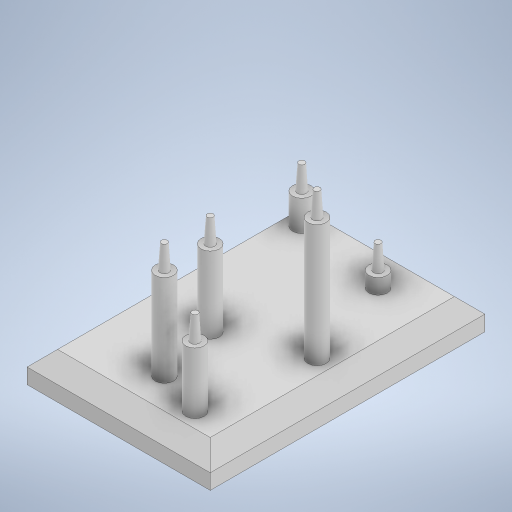
# Autodesk Inventor part: HeadTrackerProMax
Saved by Autodesk Inventor 2024 (Build 280153000, 153)
## iProperties
Created: 2024-11-04
Part Number: HeadTrackerProMax
Material: 一般
Document SubType Name: Modeling
Designer: jerry
Density: 1 g/cm^3
Appearance: 預設
Author: jerry
Autodesk Inventor part; units mm, degrees
ref_plane "YZ Plane" through (0, 0, 0) normal (1, 0, 0) x (0, 1, 0)
ref_plane "XZ Plane" through (0, 0, 0) normal (0, 1, 0) x (-1, 0, 0)
ref_plane "XY Plane" through (0, 0, 0) normal (0, 0, 1) x (1, 0, 0)
sketch "草圖1" plane through (0, 0, 0) normal (0, 1, 0) x (-1, 0, 0)
  line L0 (0, 0) -> (60, 0)
  line L1 (60, 0) -> (60, -90)
  line L2 (60, -90) -> (0, -90)
  line L3 (0, -90) -> (0, 0)
  dimension "d0" = 60
  dimension "d1" = 90
  constraints: 8 end point, 2 parallel, 1 horizontal, 1 perpendicular
  measures "d0" distance of L1.end L2.end
  measures "d1" distance of L0.end L1.end
extrude "擠出1" add sketch "草圖1" along normal blind 10
chamfer "倒角1" distance 5 angle 45 4 edges at (-60, 10, -45) (-30, 10, 0) (0, 10, -45) (-30, 10, -90)
sketch "草圖2" plane through (0, 10, 0) normal (0, 1, 0) x (1, 0, 0)
  line L0 (-60, 0) -> (0, 0) projected
  line L1 (0, 0) -> (-15, 0)
  line L2 (-15, 0) -> (-15, 10)
  line L3 (-15, 10) -> (0, 10)
  line L4 (0, 10) -> (0, 0)
  line L5 (-15, 10) -> (-30, 10)
  line L6 (-30, 10) -> (-30, 15)
  line L7 (-30, 15) -> (-15, 15)
  line L8 (-15, 15) -> (-15, 10)
  line L9 (-30, 15) -> (-35, 15)
  line L10 (-35, 15) -> (-35, 35)
  line L11 (-35, 35) -> (-30, 35)
  line L12 (-30, 35) -> (-30, 15)
  line L13 (-35, 35) -> (-50, 35)
  line L14 (-50, 35) -> (-50, 80)
  line L15 (-50, 80) -> (-35, 80)
  line L16 (-35, 80) -> (-35, 35)
  line L17 (-35, 80) -> (-20, 80)
  line L18 (-20, 80) -> (-20, 75)
  line L19 (-20, 75) -> (-35, 75)
  line L20 (-35, 75) -> (-35, 80)
  line L21 (-20, 75) -> (-10, 75)
  line L22 (-10, 75) -> (-10, 45)
  line L23 (-10, 45) -> (-20, 45)
  line L24 (-20, 45) -> (-20, 75)
  circle A0 centre (-15, 10) radius 3
  circle A1 centre (-30, 15) radius 3
  circle A2 centre (-35, 35) radius 3
  circle A3 centre (-50, 80) radius 3
  circle A4 centre (-20, 75) radius 3
  circle A5 centre (-10, 45) radius 3
  dimension "d7" = 15
  dimension "d8" = 10
  dimension "d9" = 15
  dimension "d10" = 5
  dimension "d11" = 5
  dimension "d12" = 20
  dimension "d13" = 15
  dimension "d14" = 45
  dimension "d15" = 15
  dimension "d16" = 5
  dimension "d17" = 10
  dimension "d18" = 30
  dimension "d19" = 6
  dimension "d20" = 6
  dimension "d21" = 6
  dimension "d22" = 6
  dimension "d23" = 6
  dimension "d24" = 6
  constraints: 48 end point, 12 parallel, 6 centre point, 6 coincident, 6 horizontal, 6 perpendicular
  measures "d7" distance of L2.end L3.end
  measures "d8" distance of L1.end L2.end
  measures "d9" distance of L6.end L7.end
  measures "d10" distance of L5.end L6.end
  measures "d11" distance of L11.end L10.end
  measures "d12" distance of L10.end L9.end
  measures "d13" distance of L14.end L15.end
  measures "d14" distance of L13.end L14.end
  measures "d15" distance of L18.end L19.end
  measures "d16" distance of L17.end L18.end
  measures "d17" distance of L22.end L23.end
  measures "d18" distance of L21.end L22.end
  measures "d19" diameter of A0
  measures "d20" diameter of A1
  measures "d21" diameter of A2
  measures "d22" diameter of A3
  measures "d23" diameter of A4
  measures "d24" diameter of A5
extrude "擠出2" add sketch "草圖2" along normal blind 40 contours A5 L22 L23 | L23 L22 A5
extrude "擠出3" add sketch "草圖2" along normal blind 5 contours A4 L18 L19 | L19 L24 A4 | L18 A4 L21 | L21 A4 L24
extrude "擠出4" add sketch "草圖2" along normal blind 10 contours A3 L15 L14 | L14 L15 A3
extrude "擠出5" add sketch "草圖2" along normal blind 25 contours A2 L13 L10 | L10 L11 A2 | L11 L16 A2 | L13 A2 L16
extrude "擠出6" add sketch "草圖2" along normal blind 20 contours A0 L5 L2 | L2 L3 A0 | L8 A0 L3 | L5 A0 L8
extrude "擠出7" add sketch "草圖2" along normal blind 30 contours A1 L9 L6 | L6 L7 A1 | L7 L12 A1 | L9 A1 L12
sketch "草圖3" plane through (-15, 30, -10) normal (0, 1, 0) x (1, 0, 0)
  circle A0 centre (0, 0) radius 1.5
  point P0 (15, -10)
  dimension "d37" = 3
  constraints: 1 centre point
  measures "d37" diameter of A0
sketch "草圖4" plane through (-30, 40, -15) normal (0, 1, 0) x (1, 0, 0)
  circle A0 centre (0, 0) radius 1.5
  point P0 (30, -15)
  dimension "d38" = 3
  constraints: 1 centre point
  measures "d38" diameter of A0
sketch "草圖5" plane through (-10, 50, -45) normal (0, 1, 0) x (1, 0, 0)
  circle A0 centre (0, 0) radius 1.5
  point P0 (10, -45)
  dimension "d39" = 3
  constraints: 1 centre point
  measures "d39" diameter of A0
sketch "草圖6" plane through (-35, 35, -35) normal (0, 1, 0) x (1, 0, 0)
  circle A0 centre (0, 0) radius 1.5
  point P0 (35, -35)
  dimension "d40" = 3
  constraints: 1 centre point
  measures "d40" diameter of A0
sketch "草圖7" plane through (-50, 20, -80) normal (0, 1, 0) x (1, 0, 0)
  circle A0 centre (0, 0) radius 1.5
  point P0 (50, -80)
  dimension "d41" = 3
  constraints: 1 centre point
  measures "d41" diameter of A0
sketch "草圖8" plane through (-20, 15, -75) normal (0, 1, 0) x (1, 0, 0)
  circle A0 centre (0, 0) radius 1.5
  point P0 (20, -75)
  dimension "d42" = 3
  constraints: 1 centre point
  measures "d42" diameter of A0
extrude "擠出8" add sketch "草圖8" along normal blind 8
extrude "擠出9" add sketch "草圖5" along normal blind 8
extrude "擠出10" add sketch "草圖3" along normal blind 8
extrude "擠出11" add sketch "草圖4" along normal blind 8
extrude "擠出12" add sketch "草圖6" along normal blind 8
extrude "擠出13" add sketch "草圖7" along normal blind 8
chamfer "倒角2" distance 0.5 distance2 8 1 edges at (-51.5, 28, -80) measured on face at (-50.167, 28, -80.5524)
chamfer "倒角3" distance 0.5 distance2 8 1 edges at (-21.5, 23, -75) measured on face at (-20.167, 23, -75.5524)
chamfer "倒角4" distance 0.5 distance2 8 1 edges at (-11.5, 58, -45) measured on face at (-9.1644, 58, -45.3876)
chamfer "倒角5" distance 0.5 distance2 8 1 edges at (-36.5, 43, -35) measured on face at (-34.1644, 43, -35.3876)
chamfer "倒角6" distance 0.5 distance2 8 1 edges at (-31.5, 48, -15) measured on face at (-29.1644, 48, -15.3876)
chamfer "倒角7" distance 0.5 distance2 8 1 edges at (-16.5, 38, -10) measured on face at (-14.6048, 38, -9.3766)
